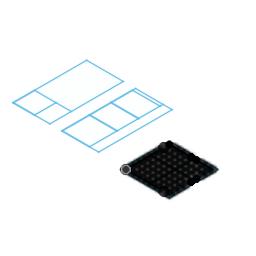
micromouse maze one quarter simpler design (Autodesk Fusion 360 design; units mm, degrees)
Autodesk Fusion 360 part; units mm, degrees
sketch "Sketch1" plane through (0, 0, 0) normal (0, 0, 1) x (1, 0, 0)
  line L0 (0, 0) -> (1440, 0)
  line L1 (1440, 0) -> (1440, 1440)
  line L2 (1440, 1440) -> (0, 1440)
  line L3 (0, 1440) -> (0, 0)
  line L4 (720, 1620) -> (720, -180)
  line L5 (0, 0) -> (180, 0)
  line L6 (180, 0) -> (180, 180)
  line L7 (180, 180) -> (0, 180)
  line L8 (0, 180) -> (0, 0)
  line L9 (0, 0) -> (0, -100)
  line L10 (0, -100) -> (-100, -100)
  line L11 (1440, 1440) -> (1540, 1440)
  line L12 (1540, 1440) -> (1540, 1540)
  dimension "d1" = 1440
  dimension "d2" = 1440
  dimension "d7" = 180
  dimension "d8" = 180
  dimension "d9" = 100
  dimension "d10" = 100
  dimension "d11" = 100
  dimension "d12" = 100
  constraint horizontal L0
  constraint vertical L1
  constraint horizontal L2
  constraint vertical L3
  constraint coincident L0.start L3.end
  constraint horizontal L5
  constraint vertical L6
  constraint horizontal L7
  constraint vertical L8
  constraint perpendicular L5 L9
  constraint perpendicular L9 L10
  constraint perpendicular L1 L11
  constraint perpendicular L11 L12
  measures "d1" distance of L0.start L0.end
  measures "d2" distance of L0.start L2.end
  measures "d7" distance of L0.start L5.end
  measures "d8" distance of L0.start L7.end
  measures "d9" distance of L0.start L9.end
  measures "d10" distance of L9.end L10.end
  measures "d11" distance of L1.end L11.end
  measures "d12" distance of L11.end L12.end
extrude "Extrude1" add sketch "Sketch1" along normal blind 12.7 makes body 1
sketch "Sketch2" plane through (0, 0, 12.7) normal (0, 0, 1) x (-1, 0, 0)
  line L0 (0, -1440) -> (0, 0)
  line L1 (0, 0) -> (-1440, 0)
  line L2 (-1440, 0) -> (-1440, -1440)
  line L3 (-1440, -1440) -> (0, -1440)
  line L4 (0, 0) -> (-180, 0)
  line L5 (-180, 0) -> (-360, 0)
  line L6 (-360, 0) -> (-540, 0)
  line L7 (-540, 0) -> (-720, 0)
  line L8 (-720, 0) -> (-720, -1440)
  line L9 (-180, 0) -> (-180, -1440)
  line L10 (-360, 0) -> (-360, -1440)
  line L11 (-540, 0) -> (-540, -1440)
  dimension "d15" = 180
  dimension "d16" = 180
  dimension "d17" = 180
  dimension "d18" = 180
  constraint coincident L0.end L1.start
  constraint perpendicular L0 L4
  constraint perpendicular L0 L5
  constraint parallel L1 L6
  constraint parallel L1 L7
  constraint midpoint L3 L8.end
  constraint coincident L3 L9.end
  constraint perpendicular L3 L9
  constraint coincident L3 L10.end
  constraint perpendicular L3 L10
  constraint coincident L3 L11.end
  constraint perpendicular L3 L11
  measures "d15" distance of L0.end L4.end
  measures "d16" distance of L4.end L5.end
  measures "d17" distance of L5.end L6.end
  measures "d18" distance of L6.end L7.end
sketch "Sketch3" plane through (0, 0, 12.7) normal (0, 0, 1) x (-1, 0, 0)
sketch "Sketch4" plane through (0, 0, 12.7) normal (0, 0, 1) x (-1, 0, 0)
  line L0 (0, 0) -> (-1440, 0)
  line L1 (-1440, 0) -> (-1440, -1440)
  line L2 (-1440, -1440) -> (0, -1440)
  line L3 (0, -1440) -> (0, 0)
  line L4 (-720, 0) -> (-810, 0)
  line L5 (-810, 0) -> (-900, 0)
  line L6 (-900, 0) -> (-1080, 0)
  line L7 (-1080, 0) -> (-1260, 0)
  line L8 (0, 0) -> (0, -180)
  line L9 (0, -180) -> (0, -360)
  line L10 (0, -360) -> (0, -540)
  line L11 (0, -540) -> (0, -720)
  line L12 (0, -720) -> (0, -900)
  line L13 (0, -900) -> (0, -1080)
  line L14 (0, -1080) -> (0, -1260)
  line L15 (-1080, 0) -> (-1260, 0)
  line L16 (0, -180) -> (0, -360)
  line L17 (-720, 0) -> (-810, 0)
  line L18 (0, -1440) -> (0, 0)
  line L19 (0, -1080) -> (0, -1260)
  line L20 (-810, 0) -> (-900, 0)
  line L21 (0, -900) -> (0, -1080)
  line L22 (0, -540) -> (0, -720)
  line L23 (-900, 0) -> (-1080, 0)
  line L24 (0, 0) -> (-1440, 0)
  line L25 (0, 0) -> (0, -180)
  line L26 (-1440, -1440) -> (0, -1440)
  line L27 (0, -720) -> (0, -900)
  line L28 (-1440, 0) -> (-1440, -1440)
  line L29 (0, -360) -> (0, -540)
  line L30 (-1080, 0) -> (-1260, 0)
  line L31 (0, -180) -> (0, -360)
  line L32 (-720, 0) -> (-810, 0)
  line L33 (0, -1440) -> (0, 0)
  line L34 (0, -1080) -> (0, -1260)
  line L35 (-810, 0) -> (-900, 0)
  line L36 (0, -900) -> (0, -1080)
  line L37 (0, -540) -> (0, -720)
  line L38 (-900, 0) -> (-1080, 0)
  line L39 (0, 0) -> (-1440, 0)
  line L40 (0, 0) -> (0, -180)
  line L41 (-1440, -1440) -> (0, -1440)
  line L42 (0, -720) -> (0, -900)
  line L43 (-1440, 0) -> (-1440, -1440)
  line L44 (0, -360) -> (0, -540)
  line L45 (0, -1440) -> (-180, -1440)
  line L46 (-180, -1440) -> (-360, -1440)
  line L47 (-360, -1440) -> (-540, -1440)
  line L48 (-540, -1440) -> (-720, -1440)
  line L49 (90, -1530) -> (-1530, -1530)
  line L50 (-1530, -1530) -> (-1530, 90)
  line L51 (-1530, 90) -> (90, 90)
  line L52 (90, 90) -> (90, -1530)
  line L53 (-720, -1440) -> (-900, -1440)
  line L54 (-1440, -720) -> (-1440, -900)
  line L55 (0, -720) -> (0, -810)
  line L56 (90, 90) -> (-824.4, 90)
  line L57 (-824.4, 90) -> (-824.4, -1530)
  line L58 (-824.4, 90) -> (-1510.2, 90)
  line L59 (90, 90) -> (90, -824.4)
  line L60 (90, -824.4) -> (-1530, -824.4)
  line L61 (2170.8056, -49.2636) -> (951.6056, -49.2636)
  line L62 (951.6056, -49.2636) -> (951.6056, -2487.6636)
  line L63 (951.6056, -2487.6636) -> (2170.8056, -2487.6636)
  line L64 (2170.8056, -2487.6636) -> (2170.8056, -49.2636)
  line L65 (2170.8056, -49.2636) -> (1256.4056, -49.2636)
  line L66 (1256.4056, -49.2636) -> (1256.4056, -963.6636)
  line L67 (1256.4056, -963.6636) -> (2170.8056, -963.6636)
  line L68 (2170.8056, -963.6636) -> (2170.8056, -49.2636)
  line L69 (2170.8056, -963.6636) -> (1256.4056, -963.6636)
  line L70 (1256.4056, -963.6636) -> (1256.4056, -1674.8636)
  line L71 (1256.4056, -1674.8636) -> (2170.8056, -1674.8636)
  line L72 (2170.8056, -1674.8636) -> (2170.8056, -963.6636)
  line L73 (2170.8056, -1674.8636) -> (1256.4056, -1674.8636)
  line L74 (1256.4056, -1674.8636) -> (1256.4056, -2386.0636)
  line L75 (1256.4056, -2386.0636) -> (2170.8056, -2386.0636)
  line L76 (2170.8056, -2386.0636) -> (2170.8056, -1674.8636)
  line L77 (3790.0355, -49.382) -> (2570.8355, -49.382)
  line L78 (2570.8355, -49.382) -> (2570.8355, -2487.782)
  line L79 (2570.8355, -2487.782) -> (3790.0355, -2487.782)
  line L80 (3790.0355, -2487.782) -> (3790.0355, -49.382)
  line L81 (3790.0355, -49.382) -> (3078.8355, -49.382)
  line L82 (3078.8355, -49.382) -> (3078.8355, -760.582)
  line L83 (3078.8355, -760.582) -> (3790.0355, -760.582)
  line L84 (3790.0355, -760.582) -> (3790.0355, -49.382)
  line L85 (1256.4056, -2386.0636) -> (1256.4056, -2487.6636)
  line L86 (3078.8355, -760.582) -> (2570.8355, -760.582)
  point P0 (0, -1440)
  point P1 (-180, -1440)
  point P2 (-360, -1440)
  point P3 (0, -1260)
  point P4 (0, -1080)
  point P5 (0, -900)
  point P6 (0, -720)
  point P7 (0, -540)
  point P8 (0, -360)
  point P9 (0, -180)
  point P10 (-180, -1260)
  point P11 (-180, -1080)
  point P12 (-180, -900)
  point P13 (-180, -720)
  point P14 (-180, -540)
  point P15 (-180, -360)
  point P16 (-180, -180)
  point P17 (-180, 0)
  point P18 (-360, -1260)
  point P19 (-360, -1080)
  point P20 (-360, -900)
  point P21 (-360, -720)
  point P22 (-360, -540)
  point P23 (-360, -360)
  point P24 (-360, -180)
  point P25 (-360, 0)
  point P26 (-540, -1440)
  point P27 (-540, -1260)
  point P28 (-540, -1080)
  point P29 (-540, -900)
  point P30 (-540, -720)
  point P31 (-540, -540)
  point P32 (-540, -360)
  point P33 (-540, -180)
  point P34 (-540, 0)
  point P35 (-720, -1440)
  point P36 (-720, -1260)
  point P37 (-720, -1080)
  point P38 (-720, -900)
  point P39 (-720, -720)
  point P40 (-720, -540)
  point P41 (-720, -360)
  point P42 (-720, -180)
  point P43 (-720, 0)
  point P44 (-900, -1440)
  point P45 (-900, -1260)
  point P46 (-900, -1080)
  point P47 (-900, -900)
  point P48 (-900, -720)
  point P49 (-900, -540)
  point P50 (-900, -360)
  point P51 (-900, -180)
  point P52 (-900, 0)
  point P53 (-1080, -1440)
  point P54 (-1080, -1260)
  point P55 (-1080, -1080)
  point P56 (-1080, -900)
  point P57 (-1080, -720)
  point P58 (-1080, -540)
  point P59 (-1080, -360)
  point P60 (-1080, -180)
  point P61 (-1080, 0)
  point P62 (-1260, -1440)
  point P63 (-1260, -1260)
  point P64 (-1260, -1080)
  point P65 (-1260, -900)
  point P66 (-1260, -720)
  point P67 (-1260, -540)
  point P68 (-1260, -360)
  point P69 (-1260, -180)
  point P70 (-1260, 0)
  point P71 (-1440, -1440)
  point P72 (-1440, -1260)
  point P73 (-1440, -1080)
  point P74 (-1440, -900)
  point P75 (-1440, -720)
  point P76 (-1440, -540)
  point P77 (-1440, -360)
  point P78 (-1440, -180)
  point P79 (-1440, 0)
  dimension "d62" = 1440
  dimension "d63" = 1440
  dimension "d86" = 914.4
  dimension "d90" = 914.4
  dimension "d92" = 1219.2
  dimension "d93" = 2438.4
  dimension "d94" = 914.4
  dimension "d95" = 914.4
  dimension "d96" = 914.4
  dimension "d97" = 711.2
  dimension "d98" = 914.4
  dimension "d99" = 711.2
  dimension "d100" = 1219.2
  dimension "d101" = 2438.4
  dimension "d102" = 711.2
  dimension "d103" = 711.2
  dimension "d105" = 180
  dimension "d106" = 180
  dimension "d107" = 1440
  dimension "d108" = 705.6
  dimension "d109" = 705.6
  constraint coincident L0.start L3.end
  constraint horizontal L0
  constraint vertical L1
  constraint horizontal L2
  constraint vertical L3
  constraint midpoint L0 P43
  constraint coincident L0 L4.end
  constraint perpendicular L0 L8
  constraint horizontal L24
  constraint vertical L28
  constraint horizontal L26
  constraint vertical L18
  constraint midpoint P43 L24
  constraint coincident L4.end L24
  constraint perpendicular L24 L25
  constraint horizontal L39
  constraint vertical L43
  constraint horizontal L41
  constraint vertical L33
  constraint midpoint L4.start L39
  constraint coincident L4.end L39
  constraint perpendicular L39 L40
  constraint perpendicular L33 L45
  constraint parallel L26 L46
  constraint parallel L41 L47
  constraint coincident P0 L2.end
  constraint horizontal L49
  constraint vertical L50
  constraint horizontal L51
  constraint vertical L52
  constraint coincident P35 L48.end
  constraint coincident P44 L53.end
  constraint coincident P75 L54.start
  constraint coincident P74 L54.end
  constraint perpendicular L32 L54
  constraint midpoint L27 L55.end
  constraint parallel L27 L55
  constraint coincident L51 L56.end
  constraint coincident L49 L57.end
  constraint perpendicular L49 L57
  constraint coincident L51 L58.end
  constraint perpendicular L51 L59
  constraint coincident L50 L60.end
  constraint perpendicular L50 L60
  constraint horizontal L61
  constraint vertical L62
  constraint horizontal L63
  constraint vertical L64
  constraint horizontal L65
  constraint vertical L66
  constraint horizontal L67
  constraint vertical L68
  constraint horizontal L69
  constraint vertical L70
  constraint horizontal L71
  constraint vertical L72
  constraint horizontal L73
  constraint vertical L74
  constraint horizontal L75
  constraint vertical L76
  constraint horizontal L77
  constraint vertical L78
  constraint horizontal L79
  constraint vertical L80
  constraint horizontal L81
  constraint vertical L82
  constraint horizontal L83
  constraint vertical L84
  constraint coincident L63 L85.end
  constraint perpendicular L63 L85
  constraint coincident L78 L86.end
  constraint perpendicular L78 L86
  measures "d86" distance of L51.end L56.end
  measures "d90" distance of L51 L60
  measures "d92" distance of L61.start L61.end
  measures "d93" distance of L61.start L63.end
  measures "d94" distance of L61.start L65.end
  measures "d95" distance of L61.start L67.end
  measures "d96" distance of L67.end L66.end
  measures "d97" distance of L67.end L71.end
  measures "d98" distance of L71.end L70.end
  measures "d99" distance of L71.end L75.end
  measures "d100" distance of L77.start L77.end
  measures "d101" distance of L77.start L79.end
  measures "d102" distance of L77.start L81.end
  measures "d103" distance of L77.start L83.end
  measures "d105" distance of P70 P79
  measures "d106" distance of P78 P79
  measures "d107" distance of P79 P71
  measures "d108" distance of L50.end L56.end
  measures "d109" distance of L49.start L59.end
sketch "Sketch6" plane through (0, 0, 12.7) normal (0, 0, 1) x (-1, 0, 0)
  line L0 (311.15, 0) -> (311.15, -2.54) construction
  line L1 (311.15, -2.54) -> (308.61, -2.54)
  line L2 (311.15, -2.54) -> (313.69, -2.54)
  line L3 (311.15, 0) -> (312.42, 0) construction
  line L4 (311.15, 0) -> (309.88, 0) construction
  line L5 (313.69, -2.54) -> (312.42, 0)
  line L6 (309.88, 0) -> (308.61, -2.54)
  line L7 (317.5, 0) -> (312.42, 0)
  line L8 (309.88, 0) -> (304.8, 0)
  line L9 (317.5, -6.35) -> (314.96, -6.35) construction
  line L10 (314.96, -6.35) -> (314.96, -8.89)
  line L11 (314.96, -6.35) -> (314.96, -3.81)
  line L12 (317.5, -6.35) -> (317.5, -7.62) construction
  line L13 (317.5, -6.35) -> (317.5, -5.08) construction
  line L14 (314.96, -3.81) -> (317.5, -5.08)
  line L15 (317.5, -7.62) -> (314.96, -8.89)
  line L16 (317.5, -7.62) -> (317.5, -12.7)
  line L17 (317.5, -5.08) -> (317.5, 0)
  line L18 (307.34, -6.35) -> (307.34, -8.89)
  line L19 (308.61, -10.16) -> (309.88, -12.7)
  line L20 (311.15, -10.16) -> (313.69, -10.16)
  line L21 (304.8, -6.35) -> (304.8, -5.08) construction
  line L22 (311.15, -12.7) -> (309.88, -12.7) construction
  line L23 (311.15, -10.16) -> (308.61, -10.16)
  line L24 (304.8, -6.35) -> (304.8, -7.62) construction
  line L25 (307.34, -6.35) -> (307.34, -3.81)
  line L26 (304.8, -6.35) -> (307.34, -6.35) construction
  line L27 (309.88, -12.7) -> (304.8, -12.7)
  line L28 (311.15, -12.7) -> (311.15, -10.16) construction
  line L29 (304.8, -5.08) -> (307.34, -3.81)
  line L30 (304.8, -12.7) -> (304.8, -7.62)
  line L31 (307.34, -8.89) -> (304.8, -7.62)
  line L32 (311.15, -12.7) -> (312.42, -12.7) construction
  line L33 (312.42, -12.7) -> (317.5, -12.7)
  line L34 (312.42, -12.7) -> (313.69, -10.16)
  line L35 (304.8, 0) -> (304.8, -5.08)
  line L36 (290.83, 0) -> (290.83, -2.54) construction
  line L37 (290.83, -2.54) -> (293.116, -2.54)
  line L38 (293.116, -2.54) -> (291.846, 0)
  line L39 (290.83, -2.54) -> (288.544, -2.54)
  line L40 (288.544, -2.54) -> (289.814, 0)
  line L41 (291.846, 0) -> (289.814, 0) construction
  line L42 (291.846, 0) -> (297.18, 0)
  line L43 (289.814, 0) -> (284.48, 0)
  line L44 (297.18, 0) -> (297.18, 1.27)
  line L45 (297.18, 1.27) -> (284.48, 1.27)
  line L46 (284.48, 1.27) -> (284.48, 0)
  dimension "d111" = 12.7
  dimension "d114" = 2.54
  dimension "d115" = 2.54
  dimension "d116" = 2.54
  dimension "d117" = 1.27
  dimension "d118" = 1.27
  dimension "d119" = 2.54
  dimension "d120" = 2.54
  dimension "d121" = 2.54
  dimension "d122" = 1.27
  dimension "d123" = 1.27
  dimension "d128" = 2.54
  dimension "d129" = 2.286
  dimension "d130" = 2.286
  dimension "d131" = 5.334
  dimension "d132" = 5.334
  dimension "d133" = 1.27
  dimension "d134" = 12.7
  constraint perpendicular L0 L1
  constraint perpendicular L0 L2
  constraint perpendicular L0 L3
  constraint perpendicular L0 L4
  constraint perpendicular L9 L10
  constraint perpendicular L9 L11
  constraint perpendicular L9 L12
  constraint perpendicular L9 L13
  constraint perpendicular L7 L17
  constraint perpendicular L8 L35
  constraint perpendicular L36 L37
  constraint perpendicular L36 L39
  constraint horizontal L41
  constraint parallel L41 L42
  constraint parallel L41 L43
  constraint perpendicular L42 L44
  constraint perpendicular L44 L45
  constraint perpendicular L43 L46
  measures "d111" distance of L8.end L7.start
  measures "d114" distance of L0.start L0.end
  measures "d115" distance of L0.end L1.end
  measures "d116" distance of L0.end L2.end
  measures "d117" distance of L0.start L3.end
  measures "d118" distance of L0.start L4.end
  measures "d119" distance of L9.start L9.end
  measures "d120" distance of L9.end L10.end
  measures "d121" distance of L9.end L11.end
  measures "d122" distance of L9.start L12.end
  measures "d123" distance of L9.start L13.end
  measures "d128" distance of L36.start L36.end
  measures "d129" distance of L36.end L37.end
  measures "d130" distance of L36.end L39.end
  measures "d131" distance of L38.end L42.end
  measures "d132" distance of L40.end L43.end
  measures "d133" distance of L42.end L44.end
  measures "d134" distance of L44.end L45.end
extrude "Extrude2" add sketch "Sketch6" along normal blind 44.45 separate body makes body 2 at (-292.9467, -1.27, 27.5167) makes body 3 at (-310.3033, 2.54, 42.3333)
sketch "Sketch7" plane through (0, 0, 57.15) normal (0, 0, 1) x (-1, 0, 0)
  line L0 (309.88, 0) -> (304.8, 0)
  line L1 (304.8, 0) -> (304.8, -5.08)
  line L2 (304.8, -5.08) -> (307.34, -3.81)
  line L3 (307.34, -3.81) -> (307.34, -8.89)
  line L4 (307.34, -8.89) -> (304.8, -7.62)
  line L5 (304.8, -7.62) -> (304.8, -12.7)
  line L6 (304.8, -12.7) -> (309.88, -12.7)
  line L7 (309.88, -12.7) -> (308.61, -10.16)
  line L8 (308.61, -10.16) -> (313.69, -10.16)
  line L9 (313.69, -10.16) -> (312.42, -12.7)
  line L10 (312.42, -12.7) -> (317.5, -12.7)
  line L11 (317.5, -12.7) -> (317.5, -7.62)
  line L12 (317.5, -7.62) -> (314.96, -8.89)
  line L13 (314.96, -8.89) -> (314.96, -3.81)
  line L14 (314.96, -3.81) -> (317.5, -5.08)
  line L15 (317.5, -5.08) -> (317.5, 0)
  line L16 (317.5, 0) -> (312.42, 0)
  line L17 (312.42, 0) -> (313.69, -2.54)
  line L18 (313.69, -2.54) -> (308.61, -2.54)
  line L19 (308.61, -2.54) -> (309.88, 0)
  line L20 (311.15, -10.16) -> (311.15, -2.54) construction
  line L21 (307.34, -6.35) -> (314.96, -6.35) construction
  circle A0 centre (311.15, -6.35) radius 3.175
  dimension "d137" = 6.35
  constraint midpoint L8 L20.start
  constraint midpoint L18 L20.end
  constraint midpoint L3 L21.start
  constraint midpoint L13 L21.end
  constraint midpoint L21 A0.centre
  measures "d137" diameter of A0
extrude "Extrude3" add sketch "Sketch7" along normal blind 12.7 contours A0 bodies 3
ref_plane "WorkPlane1" through (-311.15, 6.35, 12.7) normal (0, 0, -1) x (1, 0, 0)
sketch "Sketch8" plane through (0, 0, 12.7) normal (0, 0, -1) x (-1, 0, 0)
  line L0 (355.6, 0) -> (368.3, 12.7) construction
  line L1 (368.3, 0) -> (355.6, 12.7) construction
  circle A0 centre (361.95, 6.35) radius 3.048
  line L2 (361.95, 0) -> (364.49, 0) construction
  line L3 (359.41, 0) -> (359.41, 3.175)
  line L4 (359.41, 3.175) -> (364.49, 3.175)
  line L5 (364.49, 3.175) -> (364.49, 0)
  line L6 (368.3, 6.35) -> (368.3, 3.81) construction
  line L7 (368.3, 3.81) -> (365.125, 3.81)
  line L8 (365.125, 3.81) -> (365.125, 8.89)
  line L9 (365.125, 8.89) -> (368.3, 8.89)
  line L10 (368.3, 0) -> (368.3, 3.81)
  line L11 (368.3, 0) -> (364.49, 0)
  line L12 (359.41, 0) -> (355.6, 0)
  line L13 (368.3, 8.89) -> (368.3, 12.7)
  line L14 (359.41, 12.7) -> (359.41, 9.525)
  line L15 (364.49, 12.7) -> (368.3, 12.7)
  line L16 (355.6, 12.7) -> (359.41, 12.7)
  line L17 (355.6, 12.7) -> (355.6, 8.89)
  line L18 (364.49, 9.525) -> (364.49, 12.7)
  circle A1 centre (361.95, 6.35) radius 3.048
  line L19 (359.41, 9.525) -> (364.49, 9.525)
  line L20 (358.775, 8.89) -> (355.6, 8.89)
  line L21 (355.6, 3.81) -> (358.775, 3.81)
  line L22 (355.6, 12.7) -> (368.3, 0) construction
  line L23 (355.6, 6.35) -> (355.6, 8.89) construction
  line L24 (361.95, 12.7) -> (359.41, 12.7) construction
  line L25 (358.775, 3.81) -> (358.775, 8.89)
  line L26 (355.6, 0) -> (368.3, 12.7) construction
  line L27 (355.6, 3.81) -> (355.6, 0)
  point P0 (361.95, 6.35)
  point P1 (361.95, 6.35)
  dimension "d142" = 12.7
  dimension "d143" = 12.7
  dimension "d144" = 6.096
  dimension "d147" = 5.08
  dimension "d148" = 3.175
  dimension "d150" = 3.175
  dimension "d151" = 5.08
  constraint coincident L0 P1
  constraint coincident L1 P1
  constraint coincident P1 P0
  constraint vertical L3
  constraint horizontal L4
  constraint vertical L5
  constraint horizontal L7
  constraint vertical L8
  constraint horizontal L9
  constraint perpendicular L7 L10
  constraint perpendicular L10 L11
  constraint symmetric L12.end L0 L26.start
  constraint symmetric L1.start L0 L1.end
  constraint symmetric L13.end L0 L15.end
  constraint symmetric L1.end L0 L1.start
  constraint symmetric L0 P1 P0
  constraint symmetric L0 A0 A1
  constraint symmetric L0 L2.start L23.start
  constraint symmetric L0 L2.end L17.end
  constraint symmetric L0 L3.start L21.start
  constraint symmetric L0 L3.end L21.end
  constraint symmetric L0 L4.end L20.start
  constraint symmetric L0 L6.start L24.start
  constraint symmetric L0 L6.end L14.start
  constraint symmetric L0 L7.end L14.end
  constraint symmetric L0 L8.end L18.start
  constraint symmetric L0 L9.end L15.start
  measures "d142" distance of L0.end L1.end
  measures "d143" distance of L1.start L0.end
  measures "d144" diameter of A0
  measures "d147" distance of L2.end L3.start
  measures "d148" distance of L2.end L4.end
  measures "d150" distance of L6.end L7.end
  measures "d151" distance of L6.end L9.end
extrude "Extrude4" add sketch "Sketch8" against normal blind 57.15 separate body contours A0 A1 makes body 4
extrude "Extrude5" add sketch "Sketch8" against normal blind 44.45 bodies 4
sketch "Sketch9" plane through (0, 0, 12.7) normal (0, 0, -1) x (-1, 0, 0)
  line L0 (342.9, 0) -> (330.2, 0)
  line L1 (342.9, 0) -> (342.9, 1.27)
  line L2 (342.9, 1.27) -> (339.09, 1.27)
  line L3 (339.09, 1.27) -> (339.09, 4.445)
  line L4 (339.09, 4.445) -> (334.01, 4.445)
  line L5 (334.01, 4.445) -> (334.01, 1.27)
  line L6 (334.01, 1.27) -> (330.2, 1.27)
  line L7 (330.2, 1.27) -> (330.2, 0)
  dimension "d156" = 12.7
  dimension "d157" = 1.27
  dimension "d158" = 3.81
  dimension "d160" = 5.08
  dimension "d161" = 3.175
  constraint horizontal L0
  constraint perpendicular L0 L1
  constraint perpendicular L1 L2
  constraint perpendicular L2 L3
  constraint perpendicular L3 L4
  constraint perpendicular L4 L5
  constraint perpendicular L5 L6
  measures "d156" distance of L0.start L0.end
  measures "d157" distance of L0.start L1.end
  measures "d158" distance of L1.end L2.end
  measures "d160" distance of L3.end L4.end
  measures "d161" distance of L4.end L5.end
extrude "Extrude6" add sketch "Sketch9" against normal blind 44.45 separate body makes body 5
hidden bodies 1
equation "d111 = ( 1 / 2 ) * 1 in"
named bodies: "connector old", "post old", "post", "connector"
